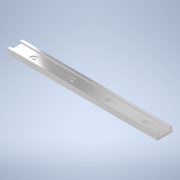
# Autodesk Inventor part: MRS20-200
Saved by Autodesk Inventor 2022 (Build 260153000, 153)
## iProperties
Created: 2022-02-08
Part Number: MRS20-200
Material: アルミニウム 6061
Document SubType Name: Modeling
Designer: satot
Density: 2.7 g/cm^3
Appearance: アルミニウム - フラット
Author: satot
Autodesk Inventor part; units mm, degrees
ref_plane "YZ Plane" through (0, 0, 0) normal (1, 0, 0) x (0, 1, 0)
ref_plane "XZ Plane" through (0, 0, 0) normal (0, 1, 0) x (-1, 0, 0)
ref_plane "XY Plane" through (0, 0, 0) normal (0, 0, 1) x (1, 0, 0)
sketch "スケッチ1" plane through (0, 0, 0) normal (0, 1, 0) x (-1, 0, 0)
  line L0 (-10, 0) -> (10, 0)
  line L1 (10, 0) -> (10, 7.2)
  line L2 (10, 7.2) -> (6.2, 7.2)
  line L3 (8.4, 3) -> (-8.4, 3)
  line L4 (-6.2, 7.2) -> (-10, 7.2)
  line L5 (-10, 7.2) -> (-10, 0)
  line L6 (6.2, 7.2) -> (6.2, 6.2)
  line L7 (6.2, 6.2) -> (8.4, 6.2)
  line L8 (8.4, 6.2) -> (8.4, 3)
  line L9 (-6.2, 7.2) -> (-6.2, 6.2)
  line L10 (-6.2, 6.2) -> (-8.4, 6.2)
  line L11 (-8.4, 6.2) -> (-8.4, 3)
  point P0 (0, 0)
  point P1 (0, 0)
  point P2 (0, 3)
  dimension "d0" = 20
  dimension "d1" = 7.2
  dimension "d2" = 3
  dimension "d3" = 12.4
  dimension "d4" = 1
  dimension "d22" = 16.8
  constraints: 25 end point, 7 perpendicular, 2 horizontal, 2 horizontal alignment, 2 midpoint, 2 vertical, 1 coincident, 1 collinear, 1 vertical alignment
  measures "d0" distance of L0.start L0.end
  measures "d1" distance of L0.end L1.end
  measures "d2" distance between parallel lines of L0 L3
  measures "d3" distance between parallel lines of L9 L6
  measures "d4" distance between parallel lines of L2 L7
  measures "d22" distance between parallel lines of L11 L8
extrude "押し出し1" add sketch "スケッチ1" along normal blind 200
chamfer "面取り1" distance 0.3 angle 45 7 edges at (-10, 100, 7.2) (-6.2, 100, 7.2) (6.2, 100, 6.2) (6.2, 100, 7.2) (10, 100, 7.2) (8.4, 100, 6.2) (-8.4, 100, 6.2)
sketch "スケッチ2" plane through (-8.4, 0, 3) normal (0, 0, 1) x (1, 0, 0)
  line L0 (0, 0) -> (16.8, 0) construction
  point P0 (8.4, 0)
  point P1 (8.4, 25)
  point P2 (8.4, 0)
  dimension "d11" = 25
  constraints: 1 midpoint, 1 vertical alignment
  measures "d11" distance from line of L0 point (8.4, 25)
hole "穴1" at (0, 25, 3) direction (0, 0, -1) diameter 4.5 end through all counterbore diameter 8.5 counterbore depth 1.8
pattern_linear "矩形状パターン1" count 10 spacing 50 along (0, 1, 0) of "穴1"
equation "\"d6\" = Length"
equation "\"Length\" = 200"
